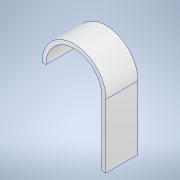
# Autodesk Inventor part: Hook 2.0
Saved by Autodesk Inventor 2020 (Build 240168000, 168)
## iProperties
Created: 2020-01-30
Part Number: Hook 2.0
Material: Aluminum 6061
Document SubType Name: Modeling
Designer: autum
Density: 2.7 g/cm^3
Appearance: Aluminum - Flat
Author: autum
Autodesk Inventor part; units mm, degrees
ref_plane "YZ Plane" through (0, 0, 0) normal (1, 0, 0) x (0, 1, 0)
ref_plane "XZ Plane" through (0, 0, 0) normal (0, 1, 0) x (-1, 0, 0)
ref_plane "XY Plane" through (0, 0, 0) normal (0, 0, 1) x (1, 0, 0)
sketch "Sketch1" plane through (0, 0, 0) normal (0, 0, 1) x (1, 0, 0)
  arc A0 (25.4, 9.8941) -> (-25.4, 9.8941) centre (0, 9.8941) ccw
  line L0 (25.4, 9.8941) -> (25.4, -40.9059)
  arc A1 (22.225, 9.8941) -> (-22.225, 9.8941) centre (0, 9.8941) ccw
  line L1 (22.225, 9.8941) -> (22.225, -40.9059)
  line L2 (22.225, -40.9059) -> (25.4, -40.9059)
  line L3 (22.225, 9.8941) -> (-22.225, 9.8941) construction
  line L4 (-25.4, 9.8941) -> (-22.225, 9.8941)
  point P0 (0, 0)
  dimension "d0" = 50.8
  dimension "d2" = 50.8
  dimension "d3" = 44.45
  constraints: 10 end point, 4 point on circle, 2 centre point, 2 coincident, 2 perpendicular, 2 tangent, 2 vertical, 1 horizontal
  measures "d0" diameter of A0
  measures "d2" distance of L0.start L0.end
  measures "d3" diameter of A1
extrude "Extrusion1" add sketch "Sketch1" along normal blind 25.4
body "Solid1"
